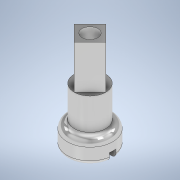
# Autodesk Inventor part: sroub
Saved by Autodesk Inventor 2022 (Build 260153000, 153)
## iProperties
Created: 2022-11-21
Part Number: sroub
Material: Generic
Document SubType Name: Modeling
Designer: matys
Density: 1 g/cm^3
Appearance: Chrome - Polished
Author: matys
Autodesk Inventor part; units mm, degrees
ref_plane "YZ Plane" through (0, 0, 0) normal (1, 0, 0) x (0, 1, 0)
ref_plane "XZ Plane" through (0, 0, 0) normal (0, 1, 0) x (-1, 0, 0)
ref_plane "XY Plane" through (0, 0, 0) normal (0, 0, 1) x (1, 0, 0)
sketch "Sketch1" plane through (0, 0, 0) normal (0, 1, 0) x (-1, 0, 0)
  circle A0 centre (0, 0) radius 2.9
  dimension "d0" = 5.8
  constraints: 1 centre point, 1 coincident
  measures "d0" diameter of A0
extrude "Extrusion1" add sketch "Sketch1" along normal blind 3
sketch "Sketch2" plane through (0, 3, 0) normal (0, 1, 0) x (1, 0, 0)
  circle A0 centre (0, 0) radius 2
  dimension "d3" = 4
  constraints: 1 centre point, 1 coincident
  measures "d3" diameter of A0
extrude "Extrusion2" add sketch "Sketch2" along normal blind 4
sketch "Sketch3" plane through (0, 7, 0) normal (0, 1, 0) x (1, 0, 0)
  circle A0 centre (0, 0) radius 2 projected
  line L0 (0, -2) -> (-2, 0)
  line L1 (-2, 0) -> (0, 2)
  line L2 (0, 2) -> (2, 0)
  line L3 (2, 0) -> (0, -2)
  constraints: 8 end point, 2 parallel, 2 point on circle, 1 perpendicular
extrude "Extrusion3" add sketch "Sketch3" along normal blind 5.5 contours L3 L0 L1 L2
fillet "Fillet1" radius 1 1 edges at (2.9, 3, 0)
fillet "Fillet2" radius 0.5 1 edges at (2.9, 0, 0)
sketch "Sketch4" plane through (0, 0, 0) normal (0, -1, 0) x (1, 0, 0)
  line L0 (0, 0) -> (-2.9, 0)
  circle A0 centre (0, 0) radius 2.9 projected
  line L1 (0, 0) -> (2.973, 0)
  line L2 (-2.9, 0.4) -> (0, 0.4)
  line L3 (0, 0.4) -> (2.973, 0.4)
  line L4 (-2.9, -0.4) -> (0, -0.4)
  line L5 (0, -0.4) -> (2.973, -0.4)
  circle A1 centre (0, 0) radius 2.9275
  point P0 (2.8723, -0.4)
  point P1 (2.8723, 0.4)
  point P2 (-2.8723, 0.4)
  point P3 (-2.8723, -0.4)
  dimension "d10" = 0.4
  dimension "d11" = 0.4
  constraints: 12 end point, 1 coincident, 1 horizontal, 1 point on line, 7 other
  measures "d10" distance between parallel lines of L1 L3
  measures "d11" distance between parallel lines of L1 L5
extrude "Extrusion4" cut sketch "Sketch4" against normal blind 1 contours L1 A0 L5 L4 L0 | L0 A0 L2 L3 L1
sketch "Sketch5" plane through (0, 12.5, 0) normal (0, 1, 0) x (1, 0, 0)
  circle A0 centre (0, 0) radius 1
  dimension "d14" = 2
  constraints: 1 centre point, 1 coincident
  measures "d14" diameter of A0
extrude "Extrusion5" cut sketch "Sketch5" against normal blind 11
body "Solid1"
